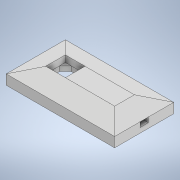
# Autodesk Inventor part: modelGatePoklice1
Saved by Autodesk Inventor 2020 (Build 240168000, 168)
## iProperties
Created: 2023-12-04
Part Number: modelGatePoklice1
Material: Generic
Document SubType Name: Sheet Metal
Designer: jirka
Density: 1 g/cm^3
Sheet Metal Rule: Default_mm
Appearance: Default
Author: jirka
Autodesk Inventor part; units mm, degrees
ref_plane "YZ Plane" through (0, 0, 0) normal (1, 0, 0) x (0, 1, 0)
ref_plane "XZ Plane" through (0, 0, 0) normal (0, 1, 0) x (-1, 0, 0)
ref_plane "XY Plane" through (0, 0, 0) normal (0, 0, 1) x (1, 0, 0)
sketch "Sketch1" plane through (0, 0, 0) normal (0, 1, 0) x (-1, 0, 0)
  line L0 (5, 5) -> (-5, 5)
  line L1 (-5, 5) -> (-5, -5)
  line L2 (-5, -5) -> (5, -5)
  line L3 (5, -5) -> (5, 5)
  line L4 (6, 6) -> (-6, 6)
  line L5 (-6, 6) -> (-6, -6)
  line L6 (-6, -6) -> (6, -6)
  line L7 (6, -6) -> (6, 6)
  point P0 (0, 0)
  dimension "d0" = 10
  dimension "d1" = 10
  dimension "d2" = 5
  dimension "d3" = 5
  dimension "d4" = 12
  dimension "d5" = 12
  dimension "d6" = 1
  dimension "d7" = 1
  constraints: 16 end point, 4 parallel, 2 horizontal, 2 perpendicular
  measures "d0" distance of L2.end L1.end
  measures "d1" distance of L1.end L0.end
  measures "d2" distance from line of point (0, 0) L3
  measures "d3" distance from line of L2 point (0, 0)
  measures "d4" distance of L6.end L5.end
  measures "d5" distance of L5.end L4.end
  measures "d6" distance between parallel lines of L7 L3
  measures "d7" distance between parallel lines of L6 L2
extrude "Extrusion1" add sketch "Sketch1" along normal blind 2
sketch "Sketch2" plane through (6, 0, 6) normal (1, 0, 0) x (0, 0, -1)
  line L0 (0, 0) -> (0, 2) projected
  line L1 (12, 0) -> (12, 2) projected
  line L2 (0, 2) -> (12, 2)
  line L3 (12, 2) -> (12, 1)
  line L4 (12, 1) -> (0, 1)
  line L5 (0, 1) -> (0, 2)
  point P0 (6, 0)
  constraints: 8 end point, 2 parallel, 1 horizontal, 1 midpoint, 1 perpendicular
extrude "Extrusion2" add sketch "Sketch2" against normal blind 11.5
sketch "Sketch3" plane through (0, 2, 0) normal (0, 1, 0) x (1, 0, 0)
  line L0 (-2, -2) -> (2, -2)
  line L1 (2, -2) -> (2, 2)
  line L2 (2, 2) -> (-2, 2)
  line L3 (-2, 2) -> (-2, -2)
  circle A0 centre (0, 0) radius 2.8284
  line L4 (0, -2.8284) -> (-2.8284, 0)
  line L5 (-2.8284, 0) -> (0, 2.8284)
  line L6 (2.8284, 0) -> (0, 2.8284)
  line L7 (2.8284, 0) -> (0, -2.8284)
  point P0 (0.8284, -2)
  point P1 (2, -0.8284)
  point P2 (2, 0.8284)
  point P3 (0.8284, 2)
  point P4 (-0.8284, 2)
  point P5 (-2, 0.8284)
  point P6 (-2, -0.8284)
  point P7 (-0.8284, -2)
  dimension "d13" = 4
  dimension "d14" = 4
  dimension "d15" = 2
  dimension "d16" = 2
  constraints: 16 end point, 5 point on circle, 4 perpendicular, 2 parallel, 1 centre point, 1 coincident, 1 horizontal
  measures "d13" distance of L1.end L2.end
  measures "d14" distance of L0.end L1.end
  measures "d15" distance from line of point (0, 0) L3
  measures "d16" distance from line of L2 point (0, 0)
extrude "Extrusion3" cut sketch "Sketch3" along normal blind 23.25 and the other way blind 11.625 contours L4 L3 L5 L2 L6 L1 L7 L0
sketch "Sketch4" plane through (0, 2, 0) normal (0, 1, 0) x (1, 0, 0)
  line L0 (2, -0.8284) -> (2, 0.8284) projected
  line L1 (2, -0.8284) -> (2.8765, -0.8284)
  line L2 (2.8765, -0.8284) -> (2.8765, 0.8284)
  line L3 (2.8765, 0.8284) -> (2, 0.8284)
  line L4 (2, 0.8284) -> (2, -0.8284)
  line L5 (2.8765, -0.8284) -> (7.5124, -0.8284)
  line L6 (7.5124, -0.8284) -> (7.5124, 0.8284)
  line L7 (7.5124, 0.8284) -> (2.8765, 0.8284)
  line L8 (2.8765, 0.8284) -> (2.8765, -0.8284)
  point P0 (0, 0)
  point P1 (2.8765, 0.8284)
  point P2 (2, 0.8284)
  constraints: 16 end point, 4 parallel, 2 horizontal, 2 perpendicular, 1 point on line
extrude "Extrusion4" cut sketch "Sketch4" against normal blind 1
sketch "Sketch5" plane through (0, 2, 0) normal (0, 1, 0) x (1, 0, 0)
  line L0 (-6, -6) -> (6, -6) projected
  line L1 (6, 0.8284) -> (6, 6) projected
  line L2 (-6, -6) -> (6, -6)
  line L3 (6, -6) -> (6, 6)
  line L4 (6, 6) -> (-6, 6)
  line L5 (-6, 6) -> (-6, -6)
  point P0 (0, 0)
  point P1 (6, -6)
  constraints: 8 end point, 2 parallel, 1 horizontal, 1 perpendicular
extrude "Extrusion5" add sketch "Sketch5" along normal blind 25
sketch "Sketch6" plane through (6, 0, 6) normal (1, 0, 0) x (0, 0, -1)
  line L0 (5.1716, 1) -> (5.1716, 2) projected
  line L1 (5.1716, 2) -> (-3.596, 2)
  line L2 (0, 0) -> (0, 27) projected
  line L3 (4, 2) -> (5.1716, 2) projected
  line L4 (5.1716, 2) -> (16.1787, 2)
  line L5 (5.1716, 2) -> (6.8284, 2) projected
  line L6 (6, 2) -> (6, 6)
  line L7 (0, 2) -> (6, 4)
  line L8 (6, 4) -> (12, 2)
  line L9 (12, 0) -> (12, 27) projected
  line L10 (12, 2) -> (-2.4689, 2)
  line L11 (-2.4689, 2) -> (-2.4689, 28.669)
  line L12 (-2.4689, 28.669) -> (12, 28.669)
  line L13 (12, 28.669) -> (12, 2)
  point P0 (6, 0)
  dimension "d23" = 4
  constraints: 18 end point, 4 point on line, 2 horizontal, 2 midpoint, 2 parallel, 2 perpendicular, 1 vertical
  measures "d23" distance of L6.start L6.end
extrude "Extrusion6" cut sketch "Sketch6" against normal blind 23.25 contours L1 L11 L12 L13 L9 L8 L7
sketch "Sketch7" plane through (-6, 0, 6) normal (0, 0, 1) x (1, 0, 0)
  line L0 (6, 0) -> (6, 4)
  line L1 (12, 4) -> (0, 4) projected
  line L2 (0, 2) -> (12, 2) projected
  line L3 (12, 2) -> (6, 4)
  line L4 (0, 4) -> (0, 2) projected
  line L5 (6, 4) -> (0, 2)
  line L6 (0, 2) -> (13.6732, 2)
  line L7 (13.6732, 2) -> (13.6732, 4.9606)
  line L8 (13.6732, 4.9606) -> (0, 4.9606)
  line L9 (0, 4.9606) -> (0, 2)
  constraints: 14 end point, 2 parallel, 1 horizontal, 1 midpoint, 1 perpendicular
extrude "Extrusion7" cut sketch "Sketch7" against normal blind 41.75 contours L5 L4 L1 | L1 L9 L8 L7 L6 L3
sketch "Sketch8" plane through (0, 2, 0) normal (0, -1, 0) x (1, 0, 0)
  line L0 (6, 6) -> (0, 0) projected
  line L1 (1.9974, 1.9974) -> (-2.0026, 1.9974)
  line L2 (-2.0026, 1.9974) -> (-2.0026, -2.0026)
  line L3 (-2.0026, -2.0026) -> (1.9974, -2.0026)
  line L4 (1.9974, -2.0026) -> (1.9974, 1.9974)
  dimension "d30" = 4
  dimension "d31" = 4
  constraints: 8 end point, 2 parallel, 1 horizontal, 1 perpendicular, 1 point on line
  measures "d30" distance of L3.end L2.end
  measures "d31" distance of L2.end L1.end
extrude "Extrusion8" cut sketch "Sketch8" against normal blind 105
sketch "Sketch9" plane through (6, 0, 6) normal (1, 0, 0) x (0, 0, -1)
  line L0 (0, 0) -> (0, 2) projected
  line L1 (12, 0) -> (12, 2) projected
  line L2 (0, 0) -> (12, 0)
  line L3 (12, 0) -> (12, 2)
  line L4 (12, 2) -> (0, 2)
  line L5 (0, 2) -> (0, 0)
  point P0 (6, 0)
  constraints: 8 end point, 2 parallel, 1 horizontal, 1 perpendicular
extrude "Extrusion9" add sketch "Sketch9" along normal blind 10
sketch "Sketch10" plane through (0, 0, 0) normal (0, -1, 0) x (1, 0, 0)
  line L0 (5, -5) -> (5, 5) projected
  line L1 (5, 5) -> (15, 5)
  line L2 (15, 5) -> (15, -5)
  line L3 (15, -5) -> (5, -5)
  line L4 (5, -5) -> (5, 5)
  point P0 (0, 0)
  dimension "d36" = 10
  constraints: 8 end point, 2 parallel, 1 horizontal, 1 perpendicular
  measures "d36" distance of L2.end L3.end
extrude "Extrusion10" cut sketch "Sketch10" against normal up to surface (1 mm away)
sketch "Sketch11" plane through (6, 2, 6) normal (0, 1, 0) x (1, 0, 0)
  line L0 (10, 0) -> (10, 12) projected
  line L1 (0, 0) -> (-4.0026, 4.0026) projected
  line L2 (10, 12) -> (-4.0026, 12)
  line L3 (-4.0026, 12) -> (-4.0026, 4.0026)
  line L4 (-4.0026, 4.0026) -> (10, 4.0026)
  line L5 (10, 4.0026) -> (10, 12)
  line L6 (-12, 0) -> (10, 0) projected
  line L7 (-4.0026, 4.0026) -> (10, 4.0026)
  line L8 (10, 4.0026) -> (10, 0)
  line L9 (10, 0) -> (-4.0026, 0)
  line L10 (-4.0026, 0) -> (-4.0026, 4.0026)
  point P0 (-6, 6)
  constraints: 16 end point, 4 parallel, 2 horizontal, 2 perpendicular
extrude "Extrusion11" add sketch "Sketch11" along normal blind 1.5 contours L6 L1 L4 L0 | L4 L3 L2 L0
sketch "Sketch12" plane through (16, 0, 6) normal (1, 0, 0) x (0, 0, -1)
  line L0 (0, 2) -> (12, 2) projected
  line L1 (4.0026, 3.3342) -> (0, 2) projected
  line L2 (4.0026, 2) -> (4.0026, 3.3342) projected
  line L3 (0, 2) -> (4.0026, 3.3342)
  line L4 (4.0026, 3.3325) -> (8.0026, 3.3325) projected
  line L5 (4.0026, 3.3342) -> (8.0026, 3.3325)
  line L6 (12, 0) -> (12, 2) projected
  line L7 (8.0026, 3.3325) -> (12, 2)
  line L8 (0, 2) -> (-1.9464, 6.2775)
  line L9 (-1.9464, 6.2775) -> (14.9869, 5.8247)
  line L10 (14.9869, 5.8247) -> (12, 2)
  point P0 (6, 0)
  constraints: 12 end point
extrude "Extrusion12" cut sketch "Sketch12" against normal blind 26 contours L8 L9 L10 L7 L4 L1
sketch "Sketch13" plane through (-6, 0, 6) normal (0, 0, 1) x (1, 0, 0)
  line L0 (3.9974, 2) -> (3.9974, 3.3325) projected
  line L1 (4.0026, 3.3342) -> (0, 2) projected
  line L2 (3.9974, 3.3325) -> (0, 3.3325)
  line L3 (0, 3.3325) -> (0, 2)
  line L4 (0, 2) -> (3.9974, 2)
  line L5 (3.9974, 2) -> (3.9974, 3.3325)
  line L6 (22, 2) -> (0, 2) projected
  line L7 (22, 3.3342) -> (4.0026, 3.3342) projected
  line L8 (22, 2) -> (18.0026, 2)
  line L9 (18.0026, 2) -> (18.0026, 3.3342)
  line L10 (18.0026, 3.3342) -> (22, 3.3342)
  line L11 (22, 3.3342) -> (22, 2)
  line L12 (18.0026, 3.3342) -> (22, 2)
  point P0 (6, 0)
  dimension "d43" = 3.9974
  dimension "d44" = 3.9974
  constraints: 18 end point, 4 parallel, 2 horizontal, 2 perpendicular, 1 point on line
  measures "d43" distance of L0.end L2.end
  measures "d44" distance between parallel lines of L11 L9
extrude "Extrusion13" cut sketch "Sketch13" against normal blind 17.75 contours L12 L7 L11
sketch "Sketch14" plane through (-5, 1, -5) normal (0, -1, 0) x (1, 0, 0)
  line L0 (11, 5.8284) -> (11, 4.1716) projected
  line L1 (11, 5.8284) -> (19.699, 5.8284)
  line L2 (19.699, 5.8284) -> (19.699, 4.1716)
  line L3 (19.699, 4.1716) -> (11, 4.1716)
  line L4 (11, 4.1716) -> (11, 5.8284)
  line L5 (19.699, 4.1716) -> (21.7329, 4.1716)
  line L6 (21.7329, 4.1716) -> (21.7329, 5.8284)
  line L7 (21.7329, 5.8284) -> (19.699, 5.8284)
  line L8 (19.699, 5.8284) -> (19.699, 4.1716)
  point P0 (5, 5)
  constraints: 16 end point, 4 parallel, 2 horizontal, 2 perpendicular, 1 point on line
extrude "Extrusion14" cut sketch "Sketch14" against normal up to surface (1 mm away)
sketch "Sketch15" plane through (0, 0, 0) normal (0, -1, 0) x (1, 0, 0)
  point P0 (0, 0)
equation "\"d2\" = 0.5 * d0"
equation "\"d3\" = 0.5 * d1"
equation "\"d15\" = 0.5 * d13"
equation "\"d16\" = 0.5 * d14"
equation "\"d44\" = d43"
equation "\"BendRadius\" = Thickness"
equation "\"BendReliefWidth\" = Thickness"
equation "\"BendReliefDepth\" = 0.5 * Thickness"
equation "\"CornerReliefSize\" = 4 * Thickness"
equation "\"MinimumRemnant\" = 2 * Thickness"
equation "\"TransitionRadius\" = BendRadius"
equation "\"JacobiRadiusSize\" = BendRadius"
equation "\"GapSize\" = Thickness"
equation "\"Thickness\" = 0.5"
body "Solid1"
